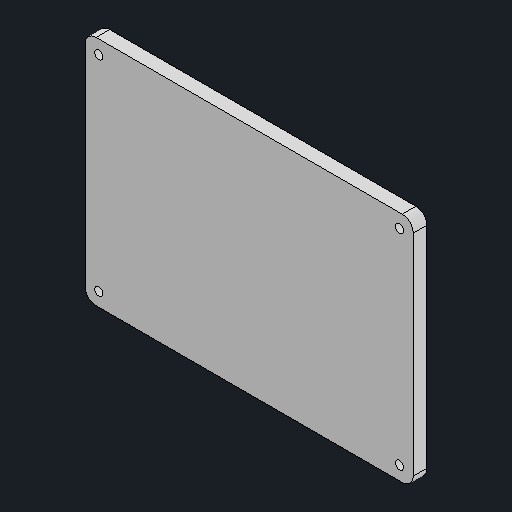
# Autodesk Inventor part: duo-esp32-pcb-outline
Saved by Autodesk Inventor 2026 (Build 300175050, 175E)
## iProperties
Created: 2025-08-22
Part Number: duo-esp32-pcb-outline
Material: Generic
Document SubType Name: Modeling
Designer: queezz
Density: 1 g/cm^3
Appearance: Default
Author: queezz
Autodesk Inventor part; units mm, degrees
ref_plane "YZ Plane" through (0, 0, 0) normal (1, 0, 0) x (0, 1, 0)
ref_plane "XZ Plane" through (0, 0, 0) normal (0, 1, 0) x (-1, 0, 0)
ref_plane "XY Plane" through (0, 0, 0) normal (0, 0, 1) x (1, 0, 0)
sketch "Sketch1" plane through (0, 0, 0) normal (0, 0, 1) x (1, 0, 0)
  line L0 (-60, 42.5) -> (60, 42.5)
  line L1 (60, 42.5) -> (60, -42.5)
  line L2 (60, -42.5) -> (-60, -42.5)
  line L3 (-60, -42.5) -> (-60, 42.5)
  point P0 (0, 0)
  point P1 (0, 42.5)
  point P2 (60, 0)
  dimension "d0" = 120
  dimension "d1" = 85
  constraints: 8 end point, 2 midpoint, 2 parallel, 1 horizontal, 1 horizontal alignment, 1 perpendicular, 1 vertical alignment
  measures "d0" distance of L0.start L0.end
  measures "d1" distance of L0.end L1.end
extrude "Extrusion1" add sketch "Sketch1" along normal blind 5
sketch "Sketch2" plane through (0, 0, 5) normal (0, 0, 1) x (1, 0, 0)
  line L0 (-55, 37.5) -> (55, 37.5) construction
  line L1 (55, 37.5) -> (55, -37.5) construction
  line L2 (55, -37.5) -> (-55, -37.5) construction
  line L3 (-55, -37.5) -> (-55, 37.5) construction
  point P0 (0, 0)
  point P1 (0, 37.5)
  point P2 (55, 0)
  point P3 (-21.4621, 82.9295)
  dimension "d4" = 110
  dimension "d5" = 75
  constraints: 8 end point, 4 coincident, 2 midpoint, 2 parallel, 1 horizontal, 1 horizontal alignment, 1 perpendicular, 1 vertical alignment
  measures "d4" distance of L0.start L0.end
  measures "d5" distance of L0.end L1.end
hole "Hole1" at (-55, 37.5, 5) at (55, 37.5, 5) at (55, -37.5, 5) at (-55, -37.5, 5) at (-21.4621, 82.9295, 5) direction (0, 0, -1) diameter 3 end through all
fillet "Fillet1" radius 4 4 edges at (60, 42.5, 2.5) (60, -42.5, 2.5) (-60, 42.5, 2.5) (-60, -42.5, 2.5)
body "Solid1"
